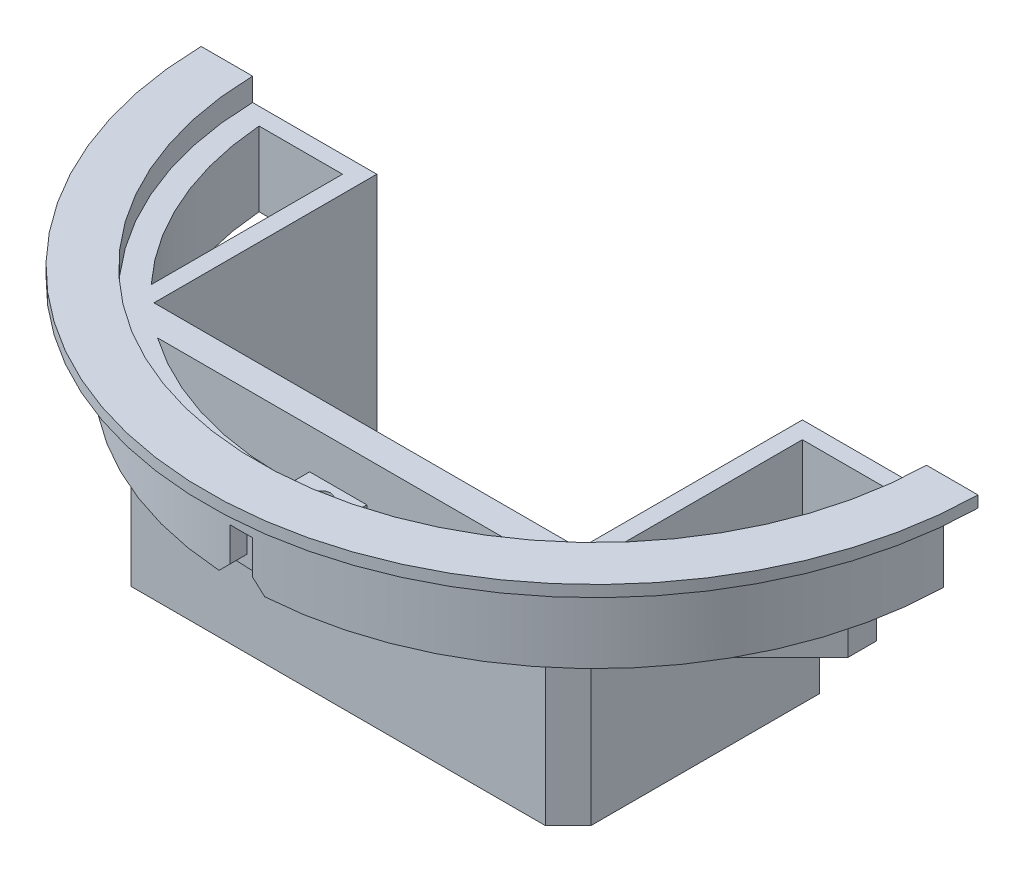
# Autodesk Inventor part: gripper_mount_female
Saved by Autodesk Inventor 2022 (Build 260153000, 153)
## iProperties
Created: 2022-03-15
Part Number: gripper_mount_female
Material: Generic
Document SubType Name: Modeling
Designer: kylem
Density: 1 g/cm^3
Appearance: Default
Author: kylem
Autodesk Inventor part; units mm, degrees
ref_plane "YZ Plane" through (0, 0, 0) normal (1, 0, 0) x (0, 1, 0)
ref_plane "XZ Plane" through (0, 0, 0) normal (0, 1, 0) x (-1, 0, 0)
sketch "Sketch1" plane through (0, 0, 0) normal (0, 1, 0) x (-1, 0, 0)
  line L0 (0, 0) -> (74.5, 0)
  line L1 (74.5, 0) -> (74.5, -40)
  line L2 (74.5, -40) -> (0, -40)
  line L3 (0, -40) -> (0, 0)
  line L4 (74.5, -40) -> (77.5, -40)
  line L5 (77.5, -40) -> (77.5, 0)
  line L6 (77.5, 0) -> (74.5, 0)
  line L7 (74.5, 0) -> (74.5, -40)
  line L8 (0, -40) -> (-3, -40)
  line L9 (-3, -40) -> (-3, 0)
  line L10 (-3, 0) -> (0, 0)
  line L11 (0, 0) -> (0, -40)
  line L12 (-3, 0) -> (77.5, 0)
  line L13 (77.5, 0) -> (77.5, 5)
  line L14 (77.5, 5) -> (-3, 5)
  line L15 (-3, 5) -> (-3, 0)
  dimension "d0" = 74.5
  dimension "d1" = 40
  dimension "d2" = 3
  dimension "d3" = 3
  dimension "d4" = 40
  dimension "d5" = 80.5
  dimension "d6" = 5
  constraints: 32 end point, 8 parallel, 4 horizontal, 4 perpendicular, 1 point on line
  measures "d0" distance of L1.end L2.end
  measures "d1" distance of L0.end L1.end
  measures "d2" distance of L6.end L5.end
  measures "d3" distance of L9.end L10.end
  measures "d4" distance of L8.end L9.end
  measures "d5" distance of L14.end L13.end
  measures "d6" distance of L13.end L12.end
extrude "Extrusion1" add sketch "Sketch1" along normal blind 40 contours L10 L15 L14 L13 L6 L0 | L3 L8 L9 L10 | L6 L5 L4 L1
sketch "Sketch3" plane through (0, 0, 0) normal (0, 0, -1) x (-1, 0, 0)
  line L0 (0, 0) -> (14.225, 0)
  line L1 (0, 0) -> (74.5, 0) projected
  line L2 (14.225, 0) -> (14.225, 8)
  circle A0 centre (14.225, 8) radius 3
  line L3 (37.25, 0) -> (37.25, 20.4526)
  line L4 (74.5, 0) -> (74.5, 40) projected
  line L5 (74.5, 0) -> (74.5, 8)
  line L6 (74.5, 8) -> (62.265, 8)
  line L7 (74.5, 8) -> (86.735, 8) construction
  circle A1 centre (62.265, 8) radius 3
  dimension "d9" = 14.225
  dimension "d10" = 8
  dimension "d11" = 6
  dimension "d12" = 8
  dimension "d13" = 12.235
  dimension "d14" = 180
  dimension "d15" = 6
  constraints: 12 end point, 2 centre point, 2 coincident, 2 perpendicular, 2 point on line, 1 collinear, 1 horizontal, 1 midpoint, 1 vertical
  measures "d9" distance of L0.start L0.end
  measures "d10" distance of L0.end L2.end
  measures "d11" diameter of A0
  measures "d12" distance of L1.end L5.end
  measures "d13" distance of L5.end L6.end
  measures "d14" angle of L6 L7
  measures "d15" diameter of A1
extrude "Extrusion2" add sketch "Sketch3" along normal blind 4
chamfer "Chamfer1" distance 1 angle 45 2 edges at (-11.225, 8, -4) (-59.265, 8, -4)
sketch "Sketch4" plane through (0, 40, 0) normal (0, 1, 0) x (1, 0, 0)
  line L0 (3, -5) -> (3, 40) projected
  line L1 (-77.5, 40) -> (-77.5, -5) projected
  line L2 (3, 40) -> (-77.5, 40)
  line L3 (-77.5, 40) -> (-77.5, 39)
  line L4 (-77.5, 39) -> (3, 39)
  line L5 (3, 39) -> (3, 40)
  point P0 (0, 0)
  dimension "d21" = 1
  constraints: 8 end point, 2 parallel, 1 horizontal, 1 perpendicular, 1 point on line
  measures "d21" distance of L3.end L2.end
extrude "Extrusion3" cut sketch "Sketch4" against normal blind 40
ref_plane "Work Plane1" through (0, 20, 0) normal (0, 1, 0) x (1, 0, 0)
sketch "Sketch6" plane through (0, 20, 0) normal (0, 1, 0) x (1, 0, 0)
  line L0 (0, 39) -> (3, 39) projected
  line L1 (3, 39) -> (13, 39)
  line L2 (13, 39) -> (13, 24)
  line L3 (13, 24) -> (3, 24)
  line L4 (3, 24) -> (3, 39)
  line L5 (0, 0) -> (-74.5, 0) projected
  line L6 (-37.25, 0) -> (-37.25, 6.791)
  line L7 (-74.5, 39) -> (-77.5, 39)
  line L8 (-77.5, 39) -> (-87.5, 39)
  line L9 (-87.5, 39) -> (-87.5, 24)
  line L10 (-87.5, 24) -> (-77.5, 24)
  line L11 (-77.5, 24) -> (-77.5, 39)
  dimension "d24" = 10
  dimension "d25" = 15
  constraints: 20 end point, 5 symmetric about line, 2 parallel, 1 horizontal, 1 midpoint, 1 perpendicular, 1 vertical
  measures "d24" distance of L2.end L3.end
  measures "d25" distance of L1.end L2.end
extrude "Extrusion4" add sketch "Sketch6" along normal mid plane 14
chamfer "Chamfer2" distance 10 angle 45 1 edges at (-87.5, 20, -24)
chamfer "Chamfer3" distance 10 angle 45 1 edges at (13, 20, -24)
sketch "Sketch7" plane through (-74.5, 40, -39) normal (0, 0, -1) x (-1, 0, 0)
  line L0 (13, -27) -> (13, -13) projected
  line L1 (3, -13) -> (13, -13) projected
  line L2 (13, -13) -> (3, -13)
  line L3 (13, -13) -> (13, -27)
  line L4 (13, -20) -> (8, -20)
  circle A0 centre (8, -20) radius 1.375
  line L5 (-74.5, 0) -> (0, 0) projected
  line L6 (-37.25, 0) -> (-37.25, -5.3996)
  circle A1 centre (-82.5, -20) radius 1.375
  point P0 (-74.5, -40)
  dimension "d34" = 5
  dimension "d35" = 2.75
  constraints: 8 end point, 2 centre point, 2 collinear, 2 midpoint, 1 coincident, 1 horizontal, 1 symmetric about line, 1 vertical, 1 other
  measures "d34" distance of L4.start L4.end
  measures "d35" diameter of A0
extrude "Extrusion5" cut sketch "Sketch7" against normal blind 14
sketch "Sketch9" plane through (0, 40, 0) normal (0, 1, 0) x (1, 0, 0)
  line L0 (-77.5, 39) -> (-77.5, -5) projected
  line L1 (13, 39) -> (3, 39) projected
  line L2 (-77.5, -5) -> (3, -5)
  line L3 (3, 39) -> (-77.5, 39)
  line L4 (-77.5, 39) -> (-77.5, -5)
  line L5 (-37.25, 39) -> (-37.25, 40)
  line L6 (-37.25, 39) -> (-36.25, 39) construction
  circle A0 centre (-37.25, 40) radius 62
  circle A1 centre (-37.25, 40) radius 55
  line L7 (-37.25, 40) -> (-42.25, 40)
  line L8 (-42.25, 40) -> (-32.25, 40)
  line L9 (-32.25, 40) -> (-32.25, -25)
  line L10 (-32.25, -25) -> (-42.25, -25)
  line L11 (-42.25, -25) -> (-42.25, 40)
  line L12 (-37.25, 39) -> (-127.25, 39)
  line L13 (-37.25, 39) -> (52.75, 39) construction
  line L14 (-127.25, 39) -> (47.7384, 39)
  line L15 (-77.5, 39) -> (-77.5, 24) projected
  line L16 (-77.5, 39) -> (-93.5, 39)
  line L17 (-93.5, 39) -> (-93.5, 36)
  line L18 (-92.1044, 36) -> (-77.5, 36)
  line L19 (-77.5, 36) -> (-77.5, 39)
  line L20 (3, -5) -> (3, 39) projected
  line L21 (3, 39) -> (19, 39)
  line L22 (19, 39) -> (19, 36)
  line L23 (17.6044, 36) -> (3, 36)
  line L24 (3, 36) -> (3, 39)
  line L25 (3, 39) -> (19, 39)
  line L26 (19, 39) -> (19, 36)
  line L27 (17.6044, 36) -> (3, 36)
  line L28 (3, 36) -> (3, 39)
  line L29 (3, -5) -> (3, 2.5175)
  line L30 (3, 36) -> (3, 39)
  point P0 (0, 0)
  point P1 (3, 2.5175)
  point P2 (-5.6272, -5)
  point P3 (-32.25, -14.7723)
  point P4 (-32.25, -5)
  point P5 (-42.25, -5)
  point P6 (-42.25, -14.7723)
  point P7 (-68.8728, -5)
  point P8 (-77.5, 2.5175)
  point P9 (-99.2419, 39)
  point P10 (24.7419, 39)
  dimension "d38" = 1
  dimension "d39" = 90
  dimension "d40" = 124
  dimension "d41" = 110
  dimension "d42" = 5
  dimension "d43" = 10
  dimension "d44" = 65
  dimension "d45" = 90
  dimension "d46" = 180
  dimension "d47" = 16
  dimension "d48" = 3
  dimension "d49" = 16
  dimension "d50" = 3
  constraints: 54 end point, 11 parallel, 8 horizontal, 6 perpendicular, 3 point on circle, 2 centre point, 2 coincident, 2 equal length, 1 collinear, 1 midpoint, 1 point on line, 1 vertical
  measures "d38" distance of L5.start L5.end
  measures "d39" angle of L6 L5
  measures "d40" diameter of A0
  measures "d41" diameter of A1
  measures "d42" distance of L7.start L7.end
  measures "d43" distance of L9.end L10.end
  measures "d44" distance of L8.end L9.end
  measures "d45" distance of L5.start L12.end
  measures "d46" angle of L12 L13
  measures "d47" distance of L18.end L17.end
  measures "d48" distance of L17.end L16.end
  measures "d49" distance of L23.end L22.end
  measures "d50" distance of L21.end L22.end
extrude "Extrusion6" add sketch "Sketch9" against normal blind 13 contours L0 L18 A1 L12 | A1 L0 L2 L11 A0 L12 | L2 L9 A1 L11 | A1 L9 A0 L11 | L14 A0 L9 A1 L2 L20 | A1 L23 L20 L1 L14
sketch "Sketch10" plane through (0, 40, 0) normal (0, 1, 0) x (1, 0, 0)
  arc A0 (-99.2419, 39) -> (24.7419, 39) centre (-37.25, 40) ccw projected
  line L0 (-37.25, -22) -> (-37.25, -10)
  circle A1 centre (-37.25, -10) radius 1.375
  point P0 (0, 0)
  dimension "d53" = 12
  dimension "d54" = 2.75
  constraints: 2 end point, 1 centre point, 1 coincident, 1 point on circle, 1 vertical
  measures "d53" distance of L0.start L0.end
  measures "d54" diameter of A1
extrude "Extrusion7" cut sketch "Sketch10" against normal blind 13
sketch "Sketch11" plane through (0, 27, 0) normal (0, -1, 0) x (1, 0, 0)
  circle A0 centre (-37.25, 10) radius 1.375 projected
  line L0 (-37.25, 10) -> (-37.25, 12)
  line L1 (-37.25, 12) -> (-37.25, 8)
  arc A1 (-38.374, 9.208) -> (-36.126, 9.208) centre (-37.25, 8) ccw
  arc A2 (-36.126, 10.792) -> (-38.374, 10.792) centre (-37.25, 12) ccw
  line L2 (-38.9, 12) -> (-38.9, 8)
  line L3 (-35.6, 8) -> (-35.6, 12)
  point P0 (0, 0)
  point P1 (-38.625, 10.25)
  point P2 (-35.875, 10.25)
  dimension "d57" = 2
  dimension "d58" = 4
  dimension "d59" = 3.3
  dimension "d60" = 3.3
  constraints: 12 point on circle, 8 end point, 3 tangent, 2 centre point, 2 coincident, 1 point on line, 1 vertical
  measures "d57" distance of L0.start L0.end
  measures "d58" distance of L0.end L1.end
  measures "d59" diameter of A1
  measures "d60" diameter of A2
extrude "Extrusion8" cut sketch "Sketch11" against normal blind 13 contours A0 A2 | A1 A0
sketch "Sketch12" plane through (0, 27, 0) normal (0, -1, 0) x (1, 0, 0)
  point P0 (0, 0)
sketch "Sketch13" plane through (0, 40, 0) normal (0, 1, 0) x (1, 0, 0)
  arc A0 (-99.2419, 39) -> (24.7419, 39) centre (-37.25, 40) ccw projected
  circle A1 centre (-37.25, 40) radius 62.25
  line L0 (-42.25, -14.7723) -> (-42.25, -5) projected
  circle A2 centre (-37.25, 40) radius 55
  line L1 (-32.25, -5) -> (-42.25, -5) projected
  line L2 (-32.25, -14.7723) -> (-32.25, -5) projected
  line L3 (-42.25, -5) -> (-32.25, -5)
  line L4 (-32.25, -5) -> (-32.25, -14.7723)
  line L5 (-42.25, -14.7723) -> (-42.25, -5)
  point P0 (0, 0)
  constraints: 6 end point, 2 centre point, 2 coincident, 1 horizontal, 1 parallel, 1 perpendicular, 1 point on circle
extrude "Extrusion9" cut sketch "Sketch13" against normal blind 7 contours L0 L1 L2 A2 picked at (-36.6938, -8.3249)
sketch "Sketch14" plane through (0, 27, 0) normal (0, -1, 0) x (1, 0, 0)
  arc A0 (-36.126, 10.792) -> (-38.374, 10.792) centre (-37.25, 12) ccw projected
  arc A1 (-35.6, 12) -> (-38.9, 12) centre (-37.25, 12) ccw
  arc A2 (-38.374, 9.208) -> (-36.126, 9.208) centre (-37.25, 8) ccw projected
  arc A3 (-38.9, 8) -> (-35.6, 8) centre (-37.25, 8) ccw
  line L0 (-35.6, 12) -> (-35.6, 8)
  line L1 (-38.9, 8) -> (-38.9, 12)
  point P0 (0, 0)
  constraints: 5 point on circle, 4 end point, 4 tangent, 2 centre point, 2 coincident, 1 parallel, 1 vertical
extrude "Extrusion10" cut sketch "Sketch14" against normal blind 10
sketch "Sketch15" plane through (0, 27, 0) normal (0, -1, 0) x (1, 0, 0)
  arc A0 (-5.6272, 5) -> (-68.8728, 5) centre (-37.25, -40) ccw projected
  line L0 (-42.25, 14.7723) -> (-42.25, 5) projected
  circle A1 centre (-37.25, -40) radius 55
  circle A2 centre (-37.25, -40) radius 62
  circle A3 centre (-37.25, -40) radius 59
  line L1 (-37.25, -40) -> (-35.25, -40)
  line L2 (-35.25, -40) -> (-39.25, -40)
  line L3 (-39.25, -40) -> (-39.25, 33.7225)
  line L4 (-39.25, 33.7225) -> (-35.25, 33.7225)
  line L5 (-35.25, 33.7225) -> (-35.25, -40)
  line L6 (-39.25, 33.7225) -> (-35.25, 33.7225)
  line L7 (-35.25, 33.7225) -> (-35.25, -40)
  line L8 (-35.25, -40) -> (-39.25, -40)
  line L9 (-39.25, -40) -> (-39.25, 33.7225)
  point P0 (0, 0)
  point P1 (-39.25, 21.9677)
  point P2 (-39.25, 18.9661)
  point P3 (-35.25, 18.9661)
  point P4 (-35.25, 21.9677)
  dimension "d67" = 118
  dimension "d68" = 2
  dimension "d69" = 4
  constraints: 18 end point, 4 parallel, 3 coincident, 3 horizontal, 2 centre point, 2 perpendicular, 3 other
  measures "d67" diameter of A3
  measures "d68" distance of L1.start L1.end
  measures "d69" distance of L3.end L4.end
extrude "Extrusion11" cut sketch "Sketch15" against normal blind 8 contours L3 A2 L5 A3 picked at (-35.6944, 19.9767)
chamfer "Chamfer4" distance 2 angle 45 2 edges at (-35.25, 27, 20.4669) (-39.25, 27, 20.4669)
sketch "Sketch16" plane through (0, 40, 0) normal (0, 1, 0) x (1, 0, 0)
  arc A0 (3, 2.5175) -> (17.6044, 36) centre (-37.25, 40) ccw projected
  circle A1 centre (-37.25, 40) radius 59
  circle A2 centre (-37.25, 40) radius 62
  line L0 (24.7419, 39) -> (0, 39) projected
  line L1 (24.7419, 39) -> (21.7415, 39)
  arc A3 (-99.2419, 39) -> (24.7419, 39) centre (-37.25, 40) ccw projected
  line L2 (-99.2419, 39) -> (-96.2415, 39)
  line L3 (-74.5, 39) -> (-99.2419, 39) projected
  point P0 (0, 0)
  dimension "d75" = 118
  constraints: 4 end point, 2 centre point, 2 coincident, 2 point on circle, 2 point on line
  measures "d75" diameter of A1
extrude "Extrusion12" add sketch "Sketch16" along normal blind 2 contours A1 L0 A2 L2 picked at (-37.25, -19.8358)
sketch "Sketch17" plane through (0, 42, 0) normal (0, 1, 0) x (1, 0, 0)
  arc A0 (-68.8728, -5) -> (-5.6272, -5) centre (-37.25, 40) ccw projected
  circle A1 centre (-37.25, 40) radius 59
  circle A2 centre (-37.25, 40) radius 68
  line L0 (3, 39) -> (13, 39) projected
  line L1 (13, 39) -> (38.5571, 39)
  line L2 (13, 39) -> (24.7419, 39) projected
  line L3 (38.5571, 39) -> (-112.8273, 39)
  point P0 (0, 0)
  point P1 (-96.2415, 39)
  point P2 (-105.2426, 39)
  point P3 (30.7426, 39)
  point P4 (21.7415, 39)
  dimension "d78" = 136
  constraints: 4 end point, 2 centre point, 2 coincident, 1 collinear, 1 point on line
  measures "d78" diameter of A2
extrude "Extrusion13" add sketch "Sketch17" along normal blind 2 contours A1 L1 A2 L3 picked at (-35.4549, -24.766)
chamfer "Chamfer5" distance 4 angle 45 2 edges at (3, 13.5, 5) (-77.5, 13.5, 5)
body "Solid1"
